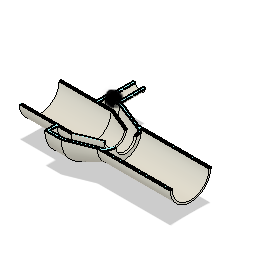
Oxygen Mixer (Autodesk Fusion 360 design; units mm, degrees)
Autodesk Fusion 360 part; units mm, degrees
sketch "Sketch7" plane through (0, 0, 0) normal (0, 1, 0) x (1, 0, 0)
  line L0 (-0.035, 8.1861) -> (9.0415, 4.4832)
  line L1 (9.0415, 4.4832) -> (8.8068, 3.9081)
  line L2 (8.8068, 3.9081) -> (-0.1031, 7.543)
  line L3 (-0.1031, 7.543) -> (-20.6566, 7.543)
  line L4 (-20.6566, 7.543) -> (-20.6566, 8.1861)
  line L5 (-5.6796, 8.1861) -> (-5.6796, 11.1664)
  line L6 (-5.6796, 11.1664) -> (-0.4049, 11.1664)
  line L7 (-0.4049, 11.1664) -> (11.7701, 6.459)
  line L8 (11.7701, 6.459) -> (12.7366, 3.7667)
  line L9 (12.7366, 3.7667) -> (13.4416, 4.0197)
  line L10 (13.4416, 4.0197) -> (12.3525, 7.0536)
  line L11 (-0.2021, 12.1178) -> (-6.7009, 12.1178)
  line L12 (-6.7009, 12.1178) -> (-6.7009, 8.1861)
  line L13 (9.9726, 8.0136) -> (38.851, 8.0136)
  line L14 (38.851, 8.0136) -> (38.851, 7.2732)
  line L15 (38.851, 7.2732) -> (11.8081, 7.2732)
  line L16 (-22.2609, 0) -> (38.4517, 0) construction
  line L17 (-20.6566, 8.1861) -> (-6.7009, 8.1861)
  line L18 (-5.6796, 8.1861) -> (-0.035, 8.1861)
  line L19 (12.3525, 7.0536) -> (11.8081, 7.2732)
  line L20 (9.9726, 8.0136) -> (-0.2021, 12.1178)
  constraint horizontal L17
  constraint perpendicular L0 L1
  constraint perpendicular L1 L2
  constraint parallel L3 L17
  constraint coincident L5.start L17
  constraint perpendicular L5 L17
  constraint perpendicular L8 L9
  constraint perpendicular L9 L10
  constraint horizontal L11
  constraint perpendicular L12 L17
  constraint coincident L13.start L19
  constraint parallel L3 L13
  constraint perpendicular L13 L14
  constraint perpendicular L14 L15
  constraint horizontal L16
  constraint coincident L16 origin
  constraint collinear L17 L18
  constraint collinear L19 L20
  constraint coincident L11.end L12.start
  constraint coincident L5.end L6.start
  constraint horizontal L6
  constraint vertical L4
revolve "Revolve1" add sketch "Sketch7" angle 360 about axis through (-22.2609, 0, 0) along (1, 0, 0) makes body 1 in component "Mixer"
ref_plane "WorkPlane4" through (-3.6451, 0, -12.1178) normal (0, 0, -1) x (0, -1, 0)
sketch "Sketch8" plane through (-3.6451, 0, -12.1178) normal (0, 0, -1) x (1, 0, 0)
  circle A0 centre (0, 0) radius 1.5
  circle A1 centre (0, 0) radius 2.5
  dimension "d17" = 3
  dimension "d19" = 1
  constraint coincident A0.centre A1.centre
  constraint concentric A0 A1
  measures "d17" diameter of A0
  measures "d19" distance of A0 A1
extrude "Extrude1" cut sketch "Sketch8" along normal up to surface contours A0 end surface at (-2.1631, -1.1118, -11.111) on bodies 1 bodies 1 in component "Mixer"
extrude "Extrude1'" add sketch "Sketch8" along normal blind 10 separate body makes body 2
copy_body "CutPasteBodies1" bodies 2 removing the originals makes body 3 in component "Mixer"
component "Mixer" placed x (1, 0, 0) y (0, 1, 0) z (0, 0, 1) at (0, 0, 0)
